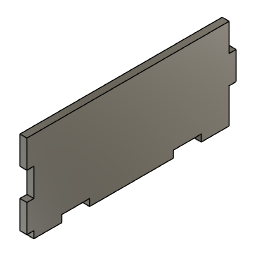
Assembly (Drawer) (Autodesk Fusion 360 archive; units mm, degrees)
design "Drawer Sides (2x)"
Autodesk Fusion 360 part; units mm, degrees
sketch "Sketch1" plane through (0, 0, 0) normal (1, 0, 0) x (0, 1, 0)
  line L0 (0, 0) -> (101.6, 0)
  line L1 (101.6, 0) -> (101.6, 38.1)
  line L2 (101.6, 38.1) -> (0, 38.1)
  line L3 (0, 38.1) -> (0, 0)
  line L4 (0, 0) -> (0, -3.175)
  line L5 (0, -3.175) -> (12.7, -3.175)
  line L6 (12.7, -3.175) -> (12.7, 0)
  line L7 (12.7, 0) -> (25.4, 0)
  line L8 (25.4, 0) -> (25.4, -3.175)
  line L9 (25.4, -3.175) -> (38.1, -3.175)
  line L10 (38.1, -3.175) -> (38.1, 0)
  line L11 (101.6, 0) -> (101.6, -3.175)
  line L12 (101.6, -3.175) -> (88.9, -3.175)
  line L13 (88.9, -3.175) -> (88.9, 0)
  line L14 (88.9, 0) -> (76.2, 0)
  line L15 (76.2, 0) -> (76.2, -3.175)
  line L16 (76.2, -3.175) -> (63.5, -3.175)
  line L17 (63.5, -3.175) -> (63.5, 0)
  line L18 (101.6, 0) -> (104.775, 0)
  line L19 (104.775, 0) -> (104.775, 12.7)
  line L20 (104.775, 12.7) -> (101.6, 12.7)
  line L21 (101.6, 38.1) -> (104.775, 38.1)
  line L22 (104.775, 38.1) -> (104.775, 25.4)
  line L23 (104.775, 25.4) -> (101.6, 25.4)
  line L24 (0, 38.1) -> (-3.175, 38.1)
  line L25 (-3.175, 38.1) -> (-3.175, 25.4)
  line L26 (-3.175, 25.4) -> (0, 25.4)
  line L27 (0, 0) -> (-3.175, 0)
  line L28 (-3.175, 0) -> (-3.175, 12.7)
  line L29 (-3.175, 12.7) -> (0, 12.7)
  dimension "d1" = 101.6
  dimension "d2" = 38.1
  dimension "d3" = 3.175
  dimension "d4" = 12.7
  dimension "d5" = 12.7
  dimension "d6" = 3.175
  dimension "d7" = 12.7
  dimension "d8" = 3.175
  dimension "d9" = 12.7
  dimension "d10" = 12.7
  dimension "d11" = 3.175
  dimension "d12" = 12.7
  dimension "d13" = 3.175
  dimension "d14" = 12.7
  dimension "d15" = 3.175
  dimension "d16" = 12.7
  dimension "d17" = 3.175
  dimension "d18" = 12.7
  dimension "d19" = 3.175
  dimension "d20" = 12.7
  constraint coincident L0.start L3.end
  constraint horizontal L0
  constraint perpendicular L0 L1
  constraint perpendicular L1 L2
  constraint perpendicular L0 L3
  constraint perpendicular L0 L4
  constraint perpendicular L4 L5
  constraint coincident L0 L6.end
  constraint perpendicular L0 L6
  constraint perpendicular L6 L7
  constraint perpendicular L0 L8
  constraint perpendicular L8 L9
  constraint coincident L0 L10.end
  constraint perpendicular L0 L10
  constraint perpendicular L0 L11
  constraint perpendicular L11 L12
  constraint coincident L0 L13.end
  constraint perpendicular L0 L13
  constraint perpendicular L13 L14
  constraint perpendicular L14 L15
  constraint perpendicular L15 L16
  constraint coincident L0 L17.end
  constraint perpendicular L0 L17
  constraint perpendicular L11 L18
  constraint perpendicular L18 L19
  constraint coincident L1 L20.end
  constraint perpendicular L1 L20
  constraint perpendicular L1 L21
  constraint perpendicular L21 L22
  constraint coincident L1 L23.end
  constraint perpendicular L1 L23
  constraint perpendicular L3 L24
  constraint perpendicular L24 L25
  constraint coincident L3 L26.end
  constraint perpendicular L3 L26
  constraint perpendicular L3 L27
  constraint perpendicular L27 L28
  constraint coincident L3 L29.end
  constraint perpendicular L3 L29
  measures "d1" distance of L0.start L0.end
  measures "d2" distance of L0.end L1.end
  measures "d3" distance of L0.start L4.end
  measures "d4" distance of L4.end L5.end
  measures "d5" distance of L6.end L7.end
  measures "d6" distance of L7.end L8.end
  measures "d7" distance of L8.end L9.end
  measures "d8" distance of L0.end L11.end
  measures "d9" distance of L11.end L12.end
  measures "d10" distance of L13.end L14.end
  measures "d11" distance of L14.end L15.end
  measures "d12" distance of L15.end L16.end
  measures "d13" distance of L0.end L18.end
  measures "d14" distance of L18.end L19.end
  measures "d15" distance of L1.end L21.end
  measures "d16" distance of L21.end L22.end
  measures "d17" distance of L2.end L24.end
  measures "d18" distance of L24.end L25.end
  measures "d19" distance of L0.start L27.end
  measures "d20" distance of L27.end L28.end
extrude "Extrude1" add sketch "Sketch1" along normal blind 3.175
sketch "Sketch2" plane through (3.175, 0, 0) normal (1, 0, 0) x (0, 1, 0)
  line L0 (0, 0) -> (0, -3.175)
  line L1 (0, -3.175) -> (12.7, -3.175)
  line L2 (12.7, -3.175) -> (12.7, 0)
  line L3 (12.7, 0) -> (25.4, 0)
  line L4 (25.4, 0) -> (25.4, -3.175)
  line L5 (25.4, -3.175) -> (38.1, -3.175)
  line L6 (38.1, -3.175) -> (38.1, 0)
  line L7 (38.1, 0) -> (63.5, 0)
  line L8 (63.5, 0) -> (63.5, -3.175)
  line L9 (63.5, -3.175) -> (76.2, -3.175)
  line L10 (76.2, -3.175) -> (76.2, 0)
  line L11 (76.2, 0) -> (88.9, 0)
  line L12 (88.9, 0) -> (88.9, -3.175)
  line L13 (88.9, -3.175) -> (101.6, -3.175)
  line L14 (101.6, -3.175) -> (101.6, 0)
  line L15 (101.6, 0) -> (104.775, 0)
  line L16 (104.775, 0) -> (104.775, 12.7)
  line L17 (104.775, 12.7) -> (101.6, 12.7)
  line L18 (101.6, 12.7) -> (101.6, 25.4)
  line L19 (101.6, 25.4) -> (104.775, 25.4)
  line L20 (104.775, 25.4) -> (104.775, 38.1)
  line L21 (104.775, 38.1) -> (-3.175, 38.1)
  line L22 (-3.175, 38.1) -> (-3.175, 25.4)
  line L23 (-3.175, 25.4) -> (0, 25.4)
  line L24 (0, 25.4) -> (0, 12.7)
  line L25 (0, 12.7) -> (-3.175, 12.7)
  line L26 (-3.175, 12.7) -> (-3.175, 0)
  line L27 (-3.175, 0) -> (0, 0)
  line L28 (50.8, 0) -> (63.5, 0)
  line L29 (63.5, 0) -> (63.5, -3.175)
  line L30 (63.5, -3.175) -> (76.2, -3.175)
  line L31 (76.2, -3.175) -> (76.2, 0)
  line L32 (76.2, 0) -> (88.9, 0)
  line L33 (88.9, -3.175) -> (88.9, 0)
  line L34 (88.9, -3.175) -> (101.6, -3.175)
  line L35 (101.6, -3.175) -> (101.6, 0)
  line L36 (104.775, 0) -> (104.775, 12.7)
  line L37 (104.775, 12.7) -> (101.6, 12.7)
  line L38 (101.6, 12.7) -> (101.6, 25.4)
  line L39 (104.775, 25.4) -> (104.775, 38.1)
  line L40 (104.775, 38.1) -> (50.8, 38.1)
  line L41 (63.5, 0) -> (57.15, 0)
  line L42 (50.8, 38.1) -> (53.975, 38.1)
  line L43 (53.975, 38.1) -> (57.15, 38.1)
  line L44 (57.15, 38.1) -> (57.15, 0)
  line L45 (57.15, 38.1) -> (57.15, 0)
  line L46 (25.4, -3.175) -> (12.7, -3.175)
  line L47 (9.525, 25.4) -> (9.525, 38.1)
  line L48 (9.525, 12.7) -> (12.7, 12.7)
  line L49 (12.7, 12.7) -> (12.7, 25.4)
  line L50 (9.525, 0) -> (9.525, 12.7)
  line L51 (12.7, -3.175) -> (12.7, 0)
  line L52 (12.7, 0) -> (9.525, 0)
  line L53 (12.7, 25.4) -> (9.525, 25.4)
  line L54 (9.525, 12.7) -> (12.7, 12.7)
  line L55 (50.8, -3.175) -> (38.1, -3.175)
  line L56 (9.525, 0) -> (9.525, 12.7)
  line L57 (9.525, 25.4) -> (9.525, 38.1)
  line L58 (38.1, 0) -> (25.4, 0)
  line L59 (38.1, -3.175) -> (38.1, 0)
  line L60 (50.8, 0) -> (50.8, -3.175)
  line L61 (12.7, -3.175) -> (12.7, 0)
  line L62 (25.4, 0) -> (25.4, -3.175)
  line L63 (50.8, 0) -> (50.8, -3.175)
  line L64 (50.8, -3.175) -> (38.1, -3.175)
  line L65 (38.1, -3.175) -> (38.1, 0)
  line L66 (25.4, -3.175) -> (25.4, 0)
  line L67 (25.4, -3.175) -> (12.7, -3.175)
  line L68 (12.7, 12.7) -> (12.7, 25.4)
  line L69 (38.1, 0) -> (25.4, 0)
  line L70 (50.8, -3.175) -> (63.5, -3.175)
  point P0 (50.8, 0)
  dimension "d23" = 3.175
  dimension "d24" = 3.175
  constraint midpoint L7 P0
  constraint coincident L7.end L8.start
  constraint coincident L8.end L9.start
  constraint coincident L9.end L10.start
  constraint coincident L10.end L11.start
  constraint coincident L11.end L12.start
  constraint coincident L12.end L13.start
  constraint coincident L13.end L14.start
  constraint coincident L14.end L15.start
  constraint coincident L15.end L16.start
  constraint coincident L16.end L17.start
  constraint coincident L17.end L18.start
  constraint coincident L18.end L19.start
  constraint coincident L19.end L20.start
  constraint coincident L20.end L21.start
  constraint midpoint L21 L40.end
  constraint midpoint L28 L41.end
  constraint parallel L40 L42
  constraint parallel L21 L43
  constraint symmetric L7.end L45 P0
  constraint symmetric L8.end L45 L55.start
  constraint symmetric L9.end L45 L5.end
  constraint symmetric L10.end L45 L6.end
  constraint symmetric L11.end L45 L3.end
  constraint symmetric L12.end L45 L4.end
  constraint symmetric L13.end L45 L1.end
  constraint symmetric L14.end L45 L2.end
  constraint symmetric L15.end L45 L50.start
  constraint symmetric L16.end L45 L48.start
  constraint symmetric L17.end L45 L48.end
  constraint symmetric L18.end L45 L49.end
  constraint symmetric L19.end L45 L47.start
  constraint symmetric L20.end L45 L47.end
  measures "d23" distance of L40.end L42.end
  measures "d24" distance of L42.end L43.end
extrude "Extrude5" add sketch "Sketch2" against normal blind 3.175 contours L6 L7 L55 L59 L60 L63 L64 L65 | L7 L8 L28 L29 L41 L60 L63 L70
extrude "Extrude3" cut sketch "Sketch2" against normal blind 30.48 contours L0 L1 L2 L21 L22 L23 L24 L25 L26 L27 L47 L48 L49 L50 L51 L52 L53 L54 L56 L57 L61 L68
extrude "Extrude2" cut sketch "Sketch2" against normal blind 15.24 contours L0 L1 L2 L21 L22 L23 L24 L25 L26 L27 L47 L48 L49 L50 L51 L52 L53 L54 L56 L57 L61 L68 | L3 L7 L21 L28 L40 L42 L43 L44 L45 L47 L48 L49 L50 L52 L53 L54 L56 L57 L58 L68 L69 | L4 L5 L6 L58 L59 L62 L65 L66 L69
extrude "Extrude4" add sketch "Sketch2" against normal blind 3.175 contours L2 L3 L4 L46 L51 L61 L62 L66 L67 | L3 L7 L21 L28 L40 L42 L43 L44 L45 L47 L48 L49 L50 L52 L53 L54 L56 L57 L58 L68 L69 | L6 L7 L55 L59 L60 L63 L64 L65
sketch "Sketch3" plane through (3.175, 0, 0) normal (1, 0, 0) x (0, 1, 0)
  line L0 (38.1, -3.175) -> (76.2, -3.175)
  line L1 (76.2, -3.175) -> (76.2, 0)
  line L2 (76.2, 0) -> (88.9, 0)
  line L3 (88.9, 0) -> (88.9, -3.175)
  line L4 (88.9, -3.175) -> (101.6, -3.175)
  line L5 (101.6, -3.175) -> (101.6, 0)
  line L6 (101.6, 0) -> (104.775, 0)
  line L7 (104.775, 0) -> (104.775, 12.7)
  line L8 (104.775, 12.7) -> (101.6, 12.7)
  line L9 (101.6, 12.7) -> (101.6, 25.4)
  line L10 (101.6, 25.4) -> (104.775, 25.4)
  line L11 (104.775, 25.4) -> (104.775, 38.1)
  line L12 (104.775, 38.1) -> (9.525, 38.1)
  line L13 (9.525, 38.1) -> (9.525, 25.4)
  line L14 (9.525, 25.4) -> (12.7, 25.4)
  line L15 (12.7, 25.4) -> (12.7, 12.7)
  line L16 (12.7, 12.7) -> (9.525, 12.7)
  line L17 (9.525, 12.7) -> (9.525, 0)
  line L18 (9.525, 0) -> (12.7, 0)
  line L19 (12.7, 0) -> (12.7, -3.175)
  line L20 (12.7, -3.175) -> (25.4, -3.175)
  line L21 (25.4, -3.175) -> (25.4, 0)
  line L22 (25.4, 0) -> (38.1, 0)
  line L23 (38.1, 0) -> (38.1, -3.175)
  line L24 (12.7, 0) -> (12.7, -3.175)
  line L25 (12.7, -3.175) -> (25.4, -3.175)
  line L26 (25.4, -3.175) -> (25.4, 0)
  line L27 (38.1, 0) -> (25.4, 0)
  line L28 (38.1, 0) -> (38.1, -3.175)
  line L29 (38.1, -3.175) -> (76.2, -3.175)
  line L30 (76.2, 0) -> (76.2, -3.175)
  line L31 (76.2, 0) -> (88.9, 0)
  line L32 (88.9, -3.175) -> (88.9, 0)
  line L33 (88.9, -3.175) -> (101.6, -3.175)
  line L34 (101.6, -3.175) -> (101.6, 0)
  line L35 (101.6, 0) -> (104.775, 0)
  line L36 (104.775, 0) -> (104.775, 12.7)
  line L37 (104.775, 12.7) -> (101.6, 12.7)
  line L38 (101.6, 12.7) -> (101.6, 25.4)
  line L39 (101.6, 25.4) -> (104.775, 25.4)
  line L40 (104.775, 25.4) -> (104.775, 38.1)
  line L41 (104.775, 38.1) -> (9.525, 38.1)
  line L42 (9.525, 38.1) -> (9.525, 25.4)
  line L43 (9.525, 25.4) -> (12.7, 25.4)
  line L44 (12.7, 25.4) -> (12.7, 12.7)
  line L45 (12.7, 12.7) -> (9.525, 12.7)
  line L46 (9.525, 12.7) -> (9.525, 0)
  line L47 (9.525, 0) -> (12.7, 0)
  constraint coincident L18.end L19.start
  constraint coincident L19.end L20.start
  constraint coincident L20.end L21.start
  constraint coincident L21.end L22.start
  constraint coincident L22.end L23.start
  constraint coincident L0.start L23.end
  constraint coincident L0.end L1.start
  constraint coincident L1.end L2.start
  constraint coincident L2.end L3.start
  constraint coincident L3.end L4.start
  constraint coincident L4.end L5.start
  constraint coincident L5.end L6.start
  constraint coincident L6.end L7.start
  constraint coincident L7.end L8.start
  constraint coincident L8.end L9.start
  constraint coincident L9.end L10.start
  constraint coincident L10.end L11.start
  constraint coincident L11.end L12.start
  constraint coincident L12.end L13.start
  constraint coincident L13.end L14.start
  constraint coincident L14.end L15.start
  constraint coincident L15.end L16.start
  constraint coincident L16.end L17.start
  constraint coincident L17.end L18.start
sketch "Sketch4" plane through (3.175, 0, 0) normal (1, 0, 0) x (0, 1, 0)
  line L0 (38.1, -3.175) -> (76.2, -3.175)
  line L1 (76.2, -3.175) -> (76.2, 0)
  line L2 (76.2, 0) -> (88.9, 0)
  line L3 (88.9, 0) -> (88.9, -3.175)
  line L4 (88.9, -3.175) -> (101.6, -3.175)
  line L5 (101.6, -3.175) -> (101.6, 0)
  line L6 (101.6, 0) -> (104.775, 0)
  line L7 (104.775, 0) -> (104.775, 12.7)
  line L8 (104.775, 12.7) -> (101.6, 12.7)
  line L9 (101.6, 12.7) -> (101.6, 25.4)
  line L10 (101.6, 25.4) -> (104.775, 25.4)
  line L11 (104.775, 25.4) -> (104.775, 38.1)
  line L12 (104.775, 38.1) -> (9.525, 38.1)
  line L13 (9.525, 38.1) -> (9.525, 25.4)
  line L14 (9.525, 25.4) -> (12.7, 25.4)
  line L15 (12.7, 25.4) -> (12.7, 12.7)
  line L16 (12.7, 12.7) -> (9.525, 12.7)
  line L17 (9.525, 12.7) -> (9.525, 0)
  line L18 (9.525, 0) -> (12.7, 0)
  line L19 (12.7, 0) -> (12.7, -3.175)
  line L20 (12.7, -3.175) -> (25.4, -3.175)
  line L21 (25.4, -3.175) -> (25.4, 0)
  line L22 (25.4, 0) -> (38.1, 0)
  line L23 (38.1, 0) -> (38.1, -3.175)
  line L24 (101.6, 12.7) -> (104.775, 12.7)
  line L25 (104.775, 25.4) -> (104.775, 12.7)
  line L26 (104.775, 25.4) -> (101.6, 25.4)
  line L27 (101.6, 25.4) -> (101.6, 12.7)
  line L28 (101.6, 25.4) -> (101.6, 38.1)
  line L29 (101.6, 38.1) -> (104.775, 38.1)
  line L30 (104.775, 38.1) -> (104.775, 0)
  line L31 (104.775, 0) -> (101.6, 0)
  line L32 (101.6, 0) -> (101.6, 25.4)
  constraint coincident L8.end L9.start
  constraint coincident L7.end L8.start
  constraint coincident L10.end L11.start
  constraint coincident L9.end L10.start
  constraint coincident L12 L28.end
  constraint perpendicular L12 L28
  constraint coincident L11.end L12.start
  constraint coincident L6.end L7.start
  constraint coincident L5.end L6.start
extrude "Extrude7" cut sketch "Sketch4" against normal blind 5.08 contours L6 L7 L8 L24 L30 L31 L32 | L10 L11 L12 L26 L28 L29 L30
extrude "Extrude6" cut sketch "Sketch4" against normal blind 20.32 contours L6 L7 L8 L24 L30 L31 L32 | L10 L11 L12 L26 L28 L29 L30
extrude "Extrude8" add sketch "Sketch4" against normal blind 3.175 contours L8 L9 L10 L24 L25 L26 L27 L30 L32

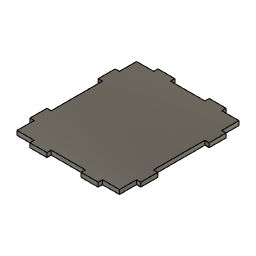
design "Drawer (bottem)"
Autodesk Fusion 360 part; units mm, degrees
sketch "Sketch1" plane through (0, 0, 0) normal (0, 0, 1) x (1, 0, 0)
  line L0 (0, 0) -> (-76.2, 0)
  line L1 (-76.2, 0) -> (-76.2, 76.2)
  line L2 (0, 76.2) -> (0, 0)
  line L3 (0, 76.2) -> (0, 88.9)
  line L4 (0, 88.9) -> (-76.2, 88.9)
  line L5 (-76.2, 88.9) -> (-76.2, 76.2)
  line L6 (-76.2, 0) -> (-63.5, 0)
  line L7 (-63.5, 0) -> (-63.5, -3.175)
  line L8 (-63.5, -3.175) -> (-50.8, -3.175)
  line L9 (-50.8, -3.175) -> (-50.8, 0)
  line L10 (-50.8, 0) -> (-38.1, 0)
  line L11 (0, 0) -> (-12.7, 0)
  line L12 (-12.7, 0) -> (-12.7, -3.175)
  line L13 (-12.7, -3.175) -> (-25.4, -3.175)
  line L14 (-25.4, -3.175) -> (-25.4, 0)
  line L15 (-76.2, 88.9) -> (-63.5, 88.9)
  line L16 (-63.5, 88.9) -> (-63.5, 92.075)
  line L17 (-63.5, 92.075) -> (-50.8, 92.075)
  line L18 (-50.8, 92.075) -> (-50.8, 88.9)
  line L19 (0, 88.9) -> (-12.7, 88.9)
  line L20 (-12.7, 88.9) -> (-12.7, 92.075)
  line L21 (-12.7, 92.075) -> (-25.4, 92.075)
  line L22 (-25.4, 92.075) -> (-25.4, 88.9)
  line L23 (-76.2, 0) -> (-76.2, 12.7)
  line L24 (-76.2, 12.7) -> (-79.375, 12.7)
  line L25 (-79.375, 12.7) -> (-79.375, 25.4)
  line L26 (-79.375, 25.4) -> (-76.2, 25.4)
  line L27 (-76.2, 88.9) -> (-76.2, 76.2)
  line L28 (-76.2, 76.2) -> (-79.375, 76.2)
  line L29 (-79.375, 76.2) -> (-79.375, 63.5)
  line L30 (-79.375, 63.5) -> (-76.2, 63.5)
  line L31 (3.175, 12.7) -> (3.175, 25.4)
  line L32 (3.175, 12.7) -> (0, 12.7)
  line L33 (3.175, 25.4) -> (0, 25.4)
  line L34 (0, 88.9) -> (0, 76.2)
  line L35 (0, 76.2) -> (3.175, 76.2)
  line L36 (3.175, 76.2) -> (3.175, 63.5)
  line L37 (3.175, 63.5) -> (0, 63.5)
  dimension "d1" = 76.2
  dimension "d2" = 76.2
  dimension "d3" = 12.7
  dimension "d4" = 3.175
  dimension "d5" = 12.7
  dimension "d6" = 12.7
  dimension "d7" = 12.7
  dimension "d8" = 3.175
  dimension "d9" = 12.7
  dimension "d10" = 12.7
  dimension "d11" = 3.175
  dimension "d12" = 12.7
  dimension "d13" = 12.7
  dimension "d14" = 3.175
  dimension "d15" = 12.7
  dimension "d16" = 12.7
  dimension "d17" = 3.175
  dimension "d18" = 12.7
  dimension "d19" = 12.7
  dimension "d20" = 3.175
  dimension "d21" = 12.7
  dimension "d24" = 12.7
  dimension "d25" = 12.7
  dimension "d26" = 3.175
  dimension "d27" = 12.7
  constraint coincident L0.start L2.end
  constraint horizontal L0
  constraint perpendicular L0 L1
  constraint perpendicular L0 L2
  constraint parallel L2 L3
  constraint perpendicular L3 L4
  constraint coincident L0 L6.end
  constraint perpendicular L6 L7
  constraint perpendicular L7 L8
  constraint coincident L0 L9.end
  constraint perpendicular L0 L9
  constraint perpendicular L9 L10
  constraint perpendicular L2 L11
  constraint perpendicular L0 L12
  constraint perpendicular L12 L13
  constraint coincident L0 L14.end
  constraint perpendicular L0 L14
  constraint perpendicular L5 L15
  constraint perpendicular L4 L16
  constraint perpendicular L16 L17
  constraint coincident L4 L18.end
  constraint perpendicular L4 L18
  constraint perpendicular L3 L19
  constraint perpendicular L4 L20
  constraint perpendicular L20 L21
  constraint coincident L4 L22.end
  constraint perpendicular L4 L22
  constraint perpendicular L0 L23
  constraint perpendicular L1 L24
  constraint perpendicular L24 L25
  constraint coincident L1 L26.end
  constraint perpendicular L1 L26
  constraint perpendicular L4 L27
  constraint perpendicular L5 L28
  constraint perpendicular L28 L29
  constraint coincident L1 L30.end
  constraint perpendicular L1 L30
  constraint coincident L2 L32.end
  constraint perpendicular L2 L32
  constraint coincident L2 L33.end
  constraint perpendicular L2 L33
  constraint perpendicular L19 L34
  constraint perpendicular L3 L35
  constraint perpendicular L35 L36
  constraint coincident L2 L37.end
  constraint perpendicular L2 L37
  measures "d1" distance of L0.start L0.end
  measures "d2" distance of L0.end L1.end
  measures "d3" distance of L2.start L3.end
  measures "d4" distance of L6.end L7.end
  measures "d5" distance of L7.end L8.end
  measures "d6" distance of L9.end L10.end
  measures "d7" distance of L0.start L11.end
  measures "d8" distance of L11.end L12.end
  measures "d9" distance of L12.end L13.end
  measures "d10" distance of L4.end L15.end
  measures "d11" distance of L15.end L16.end
  measures "d12" distance of L16.end L17.end
  measures "d13" distance of L3.end L19.end
  measures "d14" distance of L19.end L20.end
  measures "d15" distance of L20.end L21.end
  measures "d16" distance of L0.end L23.end
  measures "d17" distance of L23.end L24.end
  measures "d18" distance of L24.end L25.end
  measures "d19" distance of L4.end L1.end
  measures "d20" distance of L1.end L28.end
  measures "d21" distance of L28.end L29.end
  measures "d24" distance of L31.start L31.end
  measures "d25" distance of L3.end L2.start
  measures "d26" distance of L2.start L35.end
  measures "d27" distance of L35.end L36.end
extrude "Extrude1" add sketch "Sketch1" along normal blind 3.175

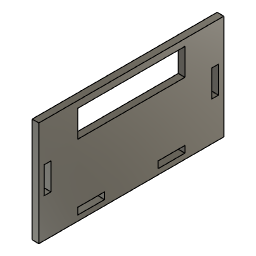
design "Drawer Front"
Autodesk Fusion 360 part; units mm, degrees
sketch "Sketch1" plane through (0, 0, 0) normal (1, 0, 0) x (0, 1, 0)
  line L0 (25.4, 0) -> (25.4, -3.175)
  line L1 (12.7, 0) -> (12.7, -3.175)
  line L2 (76.2, 25.4) -> (76.2, 12.7)
  line L3 (0, 0) -> (0, 25.4)
  line L4 (0, 12.7) -> (-3.175, 12.7)
  line L5 (76.2, 12.7) -> (79.375, 12.7)
  line L6 (-3.175, 25.4) -> (0, 25.4)
  line L7 (63.5, -3.175) -> (63.5, 0)
  line L8 (50.8, 0) -> (50.8, -3.175)
  line L9 (79.375, 12.7) -> (79.375, 25.4)
  line L10 (0, -3.175) -> (0, 0)
  line L11 (0, 0) -> (0, 12.7)
  line L12 (25.4, -3.175) -> (38.1, -3.175)
  line L13 (-3.175, 12.7) -> (-3.175, 25.4)
  line L14 (79.375, 25.4) -> (76.2, 25.4)
  line L15 (0, 0) -> (-7.62, 0)
  line L16 (0, 0) -> (-5.715, 0)
  line L17 (-5.715, 0) -> (-5.715, 38.1)
  line L18 (-5.715, 38.1) -> (-5.715, 43.815)
  line L19 (-5.715, 43.815) -> (76.2, 43.815)
  line L20 (76.2, 43.815) -> (81.915, 43.815)
  line L21 (81.915, 43.815) -> (81.915, 0)
  line L22 (81.915, 0) -> (81.915, -5.715)
  line L23 (81.915, -5.715) -> (0, -5.715)
  line L24 (0, -5.715) -> (-5.715, -5.715)
  line L25 (-5.715, -5.715) -> (-5.715, 0)
  line L26 (-5.715, 43.815) -> (12.7, 43.815)
  line L27 (12.7, 43.815) -> (12.7, 40.64)
  line L28 (12.7, 40.64) -> (12.7, 27.94)
  line L29 (81.915, 43.815) -> (63.5, 43.815)
  line L30 (63.5, 43.815) -> (63.5, 27.94)
  line L31 (63.5, 27.94) -> (12.7, 27.94)
  line L32 (12.7, 40.64) -> (63.5, 40.64)
  line L33 (63.5, -3.175) -> (50.8, -3.175)
  line L34 (63.5, 0) -> (50.8, 0)
  line L35 (25.4, -3.175) -> (12.7, -3.175)
  line L36 (12.7, 0) -> (25.4, 0)
  dimension "d2" = 12.7
  dimension "d3" = 3.175
  dimension "d4" = 12.7
  dimension "d6" = 12.7
  dimension "d9" = 12.7
  dimension "d10" = 3.175
  dimension "d12" = 12.7
  dimension "d13" = 3.175
  dimension "d14" = 12.7
  dimension "d16" = 3.175
  dimension "d17" = 12.7
  dimension "d18" = 7.62
  dimension "d21" = 5.715
  dimension "d22" = 5.715
  dimension "d23" = 5.715
  dimension "d24" = 5.715
  dimension "d25" = 3.175
  dimension "d26" = 12.7
  dimension "d27" = 18.415
  constraint coincident L3.start L10.end
  constraint perpendicular L0 L12
  constraint perpendicular L3 L4
  constraint perpendicular L4 L13
  constraint perpendicular L3 L6
  constraint perpendicular L2 L5
  constraint perpendicular L5 L9
  constraint perpendicular L2 L14
  constraint perpendicular L3 L15
  constraint perpendicular L3 L16
  constraint perpendicular L15 L17
  constraint perpendicular L15 L18
  constraint perpendicular L18 L19
  constraint perpendicular L18 L20
  constraint perpendicular L20 L21
  constraint perpendicular L20 L22
  constraint perpendicular L22 L23
  constraint perpendicular L22 L24
  constraint perpendicular L15 L25
  constraint coincident L19 L26.end
  constraint perpendicular L18 L26
  constraint perpendicular L26 L27
  constraint parallel L27 L28
  constraint perpendicular L21 L29
  constraint perpendicular L19 L30
  constraint coincident L30 L32.end
  constraint perpendicular L30 L32
  constraint perpendicular L8 L33
  constraint perpendicular L8 L34
  constraint perpendicular L1 L35
  constraint perpendicular L0 L36
  measures "d2" distance of L1.start L3.start
  measures "d3" distance of L1.start L1.end
  measures "d4" distance of L1.start L0.start
  measures "d6" distance of L0.end L12.end
  measures "d9" distance of L7.end L8.start
  measures "d10" distance of L8.start L8.end
  measures "d12" distance of L3.start L4.start
  measures "d13" distance of L4.end L4.start
  measures "d14" distance of L6.start L4.end
  measures "d16" distance of L5.end L2.end
  measures "d17" distance of L5.end L9.end
  measures "d18" distance of L3.start L15.end
  measures "d21" distance of L3.start L16.end
  measures "d22" distance of L17.end L18.end
  measures "d23" distance of L19.end L20.end
  measures "d24" distance of L21.end L22.end
  measures "d25" distance of L26.end L27.end
  measures "d26" distance of L27.end L28.end
  measures "d27" distance of L20.end L29.end
extrude "Extrude1" add sketch "Sketch1" along normal blind 3.175 contours L17 L18 L19 L20 L21 L22 L23 L24 L25 L26 L27 L28 L29 L30 L31 | L19 L27 L30 L32

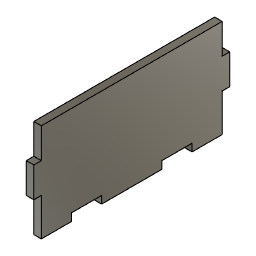
design "Drawer Back (1x)"
Autodesk Fusion 360 part; units mm, degrees
sketch "Sketch1" plane through (0, 0, 0) normal (1, 0, 0) x (0, 1, 0)
  line L0 (0, 0) -> (76.2, 0)
  line L1 (0, 0) -> (12.7, 0)
  line L2 (12.7, 0) -> (12.7, -3.175)
  line L3 (12.7, -3.175) -> (0, -3.175)
  line L4 (0, -3.175) -> (0, 0)
  line L5 (12.7, 0) -> (25.4, 0)
  line L6 (25.4, 0) -> (25.4, -3.175)
  line L7 (25.4, -3.175) -> (38.1, -3.175)
  line L8 (76.2, 0) -> (76.2, -3.175)
  line L9 (76.2, -3.175) -> (63.5, -3.175)
  line L10 (63.5, -3.175) -> (63.5, 0)
  line L11 (63.5, 0) -> (50.8, 0)
  line L12 (50.8, 0) -> (50.8, -3.175)
  line L13 (50.8, -3.175) -> (38.1, -3.175)
  line L14 (0, 0) -> (0, 38.1)
  line L15 (0, 38.1) -> (76.2, 38.1)
  line L16 (76.2, 38.1) -> (76.2, 0)
  line L17 (0, 0) -> (0, 12.7)
  line L18 (0, 12.7) -> (-3.175, 12.7)
  line L19 (-3.175, 12.7) -> (-3.175, 25.4)
  line L20 (-3.175, 25.4) -> (0, 25.4)
  line L21 (76.2, 0) -> (76.2, 12.7)
  line L22 (76.2, 12.7) -> (79.375, 12.7)
  line L23 (79.375, 12.7) -> (79.375, 25.4)
  line L24 (79.375, 25.4) -> (76.2, 25.4)
  dimension "d1" = 76.2
  dimension "d2" = 12.7
  dimension "d3" = 3.175
  dimension "d4" = 12.7
  dimension "d5" = 3.175
  dimension "d6" = 12.7
  dimension "d7" = 3.175
  dimension "d8" = 12.7
  dimension "d9" = 12.7
  dimension "d10" = 3.175
  dimension "d11" = 38.1
  dimension "d12" = 12.7
  dimension "d13" = 3.175
  dimension "d14" = 12.7
  dimension "d15" = 12.7
  dimension "d16" = 3.175
  dimension "d17" = 12.7
  constraint coincident L0.start L1.start
  constraint horizontal L0
  constraint parallel L0 L1
  constraint perpendicular L0 L2
  constraint perpendicular L2 L3
  constraint perpendicular L1 L4
  constraint perpendicular L2 L5
  constraint perpendicular L5 L6
  constraint perpendicular L6 L7
  constraint perpendicular L0 L8
  constraint perpendicular L8 L9
  constraint coincident L0 L10.end
  constraint perpendicular L0 L10
  constraint perpendicular L10 L11
  constraint perpendicular L0 L12
  constraint perpendicular L1 L14
  constraint perpendicular L14 L15
  constraint perpendicular L1 L17
  constraint perpendicular L14 L18
  constraint perpendicular L18 L19
  constraint coincident L14 L20.end
  constraint perpendicular L14 L20
  constraint perpendicular L0 L21
  constraint perpendicular L16 L22
  constraint perpendicular L22 L23
  constraint coincident L16 L24.end
  constraint perpendicular L16 L24
  measures "d1" distance of L0.start L0.end
  measures "d2" distance of L0.start L1.end
  measures "d3" distance of L1.end L2.end
  measures "d4" distance of L1.end L5.end
  measures "d5" distance of L5.end L6.end
  measures "d6" distance of L6.end L7.end
  measures "d7" distance of L0.end L8.end
  measures "d8" distance of L8.end L9.end
  measures "d9" distance of L10.end L11.end
  measures "d10" distance of L11.end L12.end
  measures "d11" distance of L0.start L14.end
  measures "d12" distance of L0.start L17.end
  measures "d13" distance of L17.end L18.end
  measures "d14" distance of L18.end L19.end
  measures "d15" distance of L0.end L21.end
  measures "d16" distance of L21.end L22.end
  measures "d17" distance of L22.end L23.end
extrude "Extrude1" add sketch "Sketch1" along normal blind 3.175
